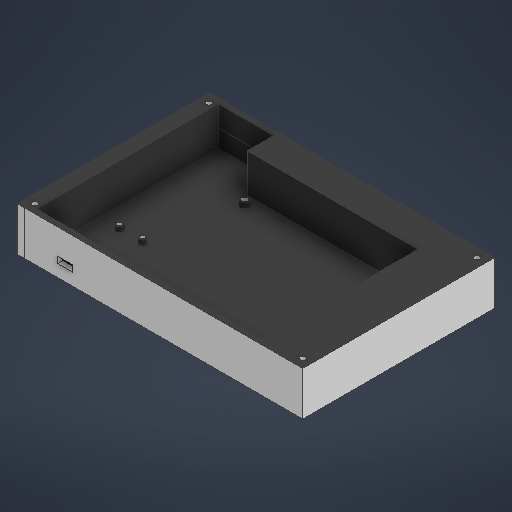
# Autodesk Inventor part: COC
Saved by Autodesk Inventor 2026 (Build 300175050, 175E)
## iProperties
Created: 2025-07-10
Part Number: COC
Material: Generic
Document SubType Name: Modeling
Designer: SaiAn
Density: 1 g/cm^3
Appearance: Default
Author: SaiAn
Autodesk Inventor part; units mm, degrees
ref_plane "YZ Plane" through (0, 0, 0) normal (1, 0, 0) x (0, 1, 0)
ref_plane "XZ Plane" through (0, 0, 0) normal (0, 1, 0) x (-1, 0, 0)
ref_plane "XY Plane" through (0, 0, 0) normal (0, 0, 1) x (1, 0, 0)
sketch "Sketch15" plane through (0, 0, 0) normal (0, 1, 0) x (-1, 0, 0)
  line L0 (0, 0) -> (97.63, 0)
  line L1 (97.63, 0) -> (97.63, -88.63)
  line L2 (97.63, -88.63) -> (0, -88.63)
  line L3 (0, -88.63) -> (0, 0)
  line L4 (-10, 10) -> (107.63, 10)
  line L5 (107.63, 10) -> (107.63, -98.63)
  line L6 (107.63, -98.63) -> (-10, -98.63)
  line L7 (-10, -98.63) -> (-10, 10)
  circle A0 centre (92.495, -6.851) radius 1.7
  circle A1 centre (93.005, -82.891) radius 1.7005
  circle A2 centre (4.245, -5.221) radius 1.7
  circle A3 centre (5.395, -84.151) radius 1.7
  circle A4 centre (92.495, -6.851) radius 2.5
  circle A5 centre (93.005, -82.891) radius 2.5
  circle A6 centre (4.245, -5.221) radius 2.5
  circle A7 centre (5.395, -84.151) radius 2.5
  dimension "d88" = 97.63
  dimension "d89" = 88.63
  dimension "d90" = 117.63
  dimension "d91" = 108.63
  dimension "d92" = 10
  dimension "d93" = 10
  dimension "d98" = 3.4
  dimension "d99" = 5.135
  dimension "d100" = 6.851
  dimension "d101" = 3.401
  dimension "d102" = 4.625
  dimension "d103" = 5.739
  dimension "d104" = 3.4
  dimension "d105" = 5.221
  dimension "d106" = 4.245
  dimension "d107" = 3.4
  dimension "d108" = 4.479
  dimension "d109" = 5.395
  dimension "d110" = 5
  dimension "d111" = 5
  dimension "d112" = 5
  dimension "d113" = 5
  constraints: 16 end point, 8 centre point, 4 coincident, 4 parallel, 2 horizontal, 2 perpendicular
  measures "d88" distance of L1.end L2.end
  measures "d89" distance of L0.end L1.end
  measures "d90" distance of L5.end L6.end
  measures "d91" distance of L4.end L5.end
  measures "d92" distance between parallel lines of L4 L0
  measures "d93" distance between parallel lines of L1 L5
  measures "d98" diameter of A0
  measures "d99" distance from line of L1 A0.centre
  measures "d100" distance from line of L0 A0.centre
  measures "d101" diameter of A1
  measures "d102" distance from line of L1 A1.centre
  measures "d103" distance from line of L2 A1.centre
  measures "d104" diameter of A2
  measures "d105" distance from line of L0 A2.centre
  measures "d106" distance from line of L3 A2.centre
  measures "d107" diameter of A3
  measures "d108" distance from line of L2 A3.centre
  measures "d109" distance from line of L3 A3.centre
  measures "d110" diameter of A4
  measures "d111" diameter of A5
  measures "d112" diameter of A6
  measures "d113" diameter of A7
extrude "Extrusion21" add sketch "Sketch15" along normal blind 3 contours L0 L1 L2 L3 | A0 | A1 | A2 | A3 | A4 | A5 | A6 | A7
extrude "Extrusion22" add sketch "Sketch15" along normal blind 13 contours L4 L5 L6 L7
extrude "Extrusion23" cut sketch "Sketch15" along normal blind 13 contours A0 | A1 | A2 | A3
extrude "Extrusion24" add sketch "Sketch15" along normal blind 6 contours A4 | A5 | A6 | A7
sketch "Sketch16" plane through (10, 0, -98.63) normal (0, 0, -1) x (-1, 0, 0)
  line L0 (0, 13) -> (117.63, 13) projected
  line L1 (117.63, 0) -> (0, 0) projected
  line L2 (117.63, 13) -> (0, 13)
  line L3 (0, 13) -> (0, 0)
  line L4 (0, 0) -> (117.63, 0)
  line L5 (117.63, 0) -> (117.63, 13)
  point P0 (10, 0)
  constraints: 8 end point, 2 parallel, 1 horizontal, 1 perpendicular
extrude "Extrusion25" add sketch "Sketch16" along normal blind 15.696
sketch "Sketch17" plane through (-97.63, 3, -88.63) normal (1, 0, 0) x (0, 0, -1)
  line L0 (0, 0) -> (0, 10) projected
  line L1 (-88.63, 10) -> (0, 10)
  line L2 (0, 10) -> (0, 0)
  line L3 (0, 0) -> (-88.63, 0)
  line L4 (-88.63, 0) -> (-88.63, 10)
  point P0 (-88.63, -3)
  constraints: 8 end point, 2 parallel, 1 horizontal, 1 perpendicular
extrude "Extrusion26" cut sketch "Sketch17" against normal blind 10
sketch "Sketch18" plane through (-107.63, 0, 10) normal (-1, 0, 0) x (0, 0, 1)
  line L0 (-98.63, 13) -> (-124.326, 13) projected
  line L1 (-124.326, 13) -> (-124.326, 0)
  line L2 (-124.326, 0) -> (0.0056, 0)
  line L3 (0.0056, 0) -> (0.0056, 13.0075)
  line L4 (0.0056, 13.0075) -> (-10, 13.0075)
  line L5 (-10, 13.0075) -> (-10, 3)
  line L6 (-98.63, 3) -> (-98.63, 13) projected
  line L7 (-10, 3) -> (-98.63, 3)
  line L8 (-98.63, 3) -> (-98.63, 13)
  point P0 (-10, 0)
  constraints: 14 end point, 6 perpendicular, 1 vertical
extrude "Extrusion27" add sketch "Sketch18" along normal blind 25
sketch "Sketch19" plane through (0, 3, 0) normal (0, 0, -1) x (-1, 0, 0)
  line L0 (107.63, 10.0075) -> (132.63, 10.0075) projected
  line L1 (132.63, 0) -> (0, 0) projected
  line L2 (132.63, 10.0075) -> (122.63, 10.0075)
  line L3 (122.63, 10.0075) -> (122.63, 0)
  line L4 (122.63, 0) -> (132.63, 0)
  line L5 (132.63, 0) -> (132.63, 10.0075)
  point P0 (0, -3)
  dimension "d124" = 10
  constraints: 8 end point, 2 parallel, 1 horizontal, 1 perpendicular, 1 point on line
  measures "d124" distance of L4.end L3.end
extrude "Extrusion28" add sketch "Sketch19" along normal blind 88.63
sketch "Sketch20" plane through (0, 3, 0) normal (0, 1, 0) x (1, 0, 0)
  circle A0 centre (-118.282, 3.585) radius 1.25
  line L0 (-107.63, 0) -> (-122.63, 0) projected
  line L1 (-122.63, 0) -> (-122.63, 88.63) projected
  circle A1 centre (-118.282, 3.585) radius 2
  circle A2 centre (-100.632, 3.585) radius 1.25
  circle A3 centre (-100.632, 3.585) radius 2
  circle A4 centre (-103.397, 35.123) radius 1.25
  line L2 (0, 0) -> (-107.63, 0) projected
  circle A5 centre (-116.397, 35.123) radius 1.25
  circle A6 centre (-103.397, 35.123) radius 2
  circle A7 centre (-116.397, 35.123) radius 2
  dimension "d127" = 2.5
  dimension "d128" = 3.585
  dimension "d129" = 4.348
  dimension "d130" = 4
  dimension "d131" = 2.5
  dimension "d132" = 3.585
  dimension "d133" = 21.998
  dimension "d134" = 4
  dimension "d135" = 2.5
  dimension "d136" = 19.233
  dimension "d137" = 35.123
  dimension "d138" = 2.5
  dimension "d139" = 6.233
  dimension "d140" = 35.123
  dimension "d141" = 4
  dimension "d142" = 4
  constraints: 8 centre point, 4 coincident
  measures "d127" diameter of A0
  measures "d128" distance from line of L0 A0.centre
  measures "d129" distance from line of L1 A0.centre
  measures "d130" diameter of A1
  measures "d131" diameter of A2
  measures "d132" distance from line of L0 A2.centre
  measures "d133" distance from line of L1 A2.centre
  measures "d134" diameter of A3
  measures "d135" diameter of A4
  measures "d136" distance from line of L1 A4.centre
  measures "d137" distance from line of L2 A4.centre
  measures "d138" diameter of A5
  measures "d139" distance from line of L1 A5.centre
  measures "d140" distance from line of L0 A5.centre
  measures "d141" diameter of A6
  measures "d142" diameter of A7
extrude "Extrusion29" add sketch "Sketch20" along normal blind 3
extrude "Extrusion30" cut sketch "Sketch20" against normal blind 6 contours A0 | A2 | A4 | A5
sketch "Sketch21" plane through (-122.63, 3, 0) normal (1, 0, 0) x (0, 0, -1)
  line L0 (88.63, 10) -> (88.63, 0) projected
  line L1 (0, 10.0075) -> (88.63, 10.0075) projected
  line L2 (88.63, 0) -> (0, 0)
  line L3 (0, 0) -> (0, 10.0075)
  line L4 (0, 10.0075) -> (88.63, 10.0075)
  line L5 (88.63, 10.0075) -> (88.63, 0)
  point P0 (0, -3)
  constraints: 8 end point, 2 parallel, 1 horizontal, 1 perpendicular
extrude "Extrusion31" cut sketch "Sketch21" against normal blind 6
sketch "Sketch22" plane through (0, 3, -88.63) normal (0, 0, 1) x (1, 0, 0)
  line L0 (0, 0) -> (-128.63, 0) projected
  line L1 (-128.63, 10) -> (0, 10) projected
  line L2 (-128.63, 0) -> (-97.315, 0)
  line L3 (-97.315, 0) -> (-97.315, 10)
  line L4 (-97.315, 10) -> (-128.63, 10)
  line L5 (-128.63, 10) -> (-128.63, 0)
  point P0 (0, -3)
  dimension "d149" = 31.315
  constraints: 8 end point, 2 parallel, 1 horizontal, 1 perpendicular, 1 point on line
  measures "d149" distance of L4.end L3.end
extrude "Extrusion32" cut sketch "Sketch22" against normal blind 15
sketch "Sketch23" plane through (10, 0, 10) normal (1, 0, 0) x (0, 0, -1)
  line L0 (0, 13) -> (10, 13) projected
  line L1 (124.326, 0) -> (-0.0056, 0) projected
  line L2 (0, 13) -> (124.326, 13)
  line L3 (124.326, 13) -> (124.326, 0)
  line L4 (124.326, 0) -> (0, 0)
  line L5 (0, 0) -> (0, 13)
  point P0 (10, 0)
  point P1 (0, 0)
  constraints: 8 end point, 2 parallel, 1 horizontal, 1 perpendicular
extrude "Extrusion33" add sketch "Sketch23" along normal blind 20
sketch "Sketch24" plane through (0, 13, 0) normal (0, 1, 0) x (1, 0, 0)
  line L0 (-107.63, -10) -> (30, -10) projected
  line L1 (30, 114.326) -> (14, 114.326)
  line L2 (14, 114.326) -> (14, -10)
  line L3 (14, -10) -> (30, -10)
  line L4 (30, -10) -> (30, 114.326)
  point P0 (0, 0)
  dimension "d154" = 16
  constraints: 8 end point, 2 parallel, 1 horizontal, 1 perpendicular, 1 point on line
  measures "d154" distance of L3.end L2.end
extrude "Extrusion34" add sketch "Sketch24" along normal blind 12
sketch "Sketch25" plane through (0, 13, 0) normal (0, 1, 0) x (1, 0, 0)
  line L0 (14, 114.326) -> (-132.63, 114.326) projected
  line L1 (-107.63, -10) -> (14, -10) projected
  line L2 (14, 114.326) -> (0, 114.326)
  line L3 (0, 114.326) -> (0, -10)
  line L4 (0, -10) -> (14, -10)
  line L5 (14, -10) -> (14, 114.326)
  line L6 (0, 88.63) -> (-97.315, 88.63) projected
  line L7 (0, 114.326) -> (-97.315, 114.326)
  line L8 (-97.315, 114.326) -> (-97.315, 88.63)
  line L9 (-97.315, 88.63) -> (0, 88.63)
  line L10 (0, 88.63) -> (0, 114.326)
  line L11 (0, 0) -> (-107.63, 0) projected
  line L12 (0, 0) -> (-132.63, 0)
  line L13 (-132.63, 0) -> (-132.63, -10)
  line L14 (-132.63, -10) -> (0, -10)
  line L15 (0, -10) -> (0, 0)
  line L16 (-107.63, 0) -> (-128.63, 0) projected
  line L17 (-128.63, 0) -> (-132.63, 0)
  line L18 (-132.63, 0) -> (-132.63, 114.326)
  line L19 (-132.63, 114.326) -> (-128.63, 114.326)
  line L20 (-128.63, 114.326) -> (-128.63, 0)
  line L21 (-97.315, 114.326) -> (-128.63, 114.326)
  line L22 (-128.63, 114.326) -> (-128.63, 103.6198)
  line L23 (-128.63, 103.6198) -> (-97.315, 103.6198)
  line L24 (-97.315, 103.6198) -> (-97.315, 114.326)
  point P0 (14, -10)
  constraints: 40 end point, 10 parallel, 5 horizontal, 5 perpendicular, 3 point on line
extrude "Extrusion35" add sketch "Sketch25" along normal blind 12 contours L5 L1 L3 L0 | L3 L6 L8 L0 | L8 L23 L20 L0 | L1 L14 L13 L12 L11 L3 | L20 L12 L18 L0
sketch "Sketch26" plane through (10, 0, -114.326) normal (0, 0, -1) x (-1, 0, 0)
  line L0 (-20, 0) -> (-20, 25) projected
  line L1 (-20, 0) -> (142.4813, 0)
  line L2 (142.4813, 0) -> (142.4813, 25)
  line L3 (142.4813, 25) -> (-20, 25)
  line L4 (-20, 25) -> (-20, 0)
  point P0 (10, 0)
  constraints: 8 end point, 2 parallel, 1 horizontal, 1 perpendicular
extrude "Extrusion36" cut sketch "Sketch26" against normal blind 8
sketch "Sketch27" plane through (-132.4813, 0, -114.326) normal (1, 0, 0) x (0, 0, -1)
  line L0 (0, 25) -> (-124.326, 25) projected
  line L1 (0, 0) -> (-7.9474, 0)
  line L2 (-7.9474, 0) -> (-7.9474, 25)
  line L3 (-7.9474, 25) -> (0, 25)
  line L4 (0, 25) -> (0, 0)
  point P0 (-114.326, 0)
  constraints: 8 end point, 2 parallel, 1 horizontal, 1 perpendicular, 1 point on line
extrude "Extrusion37" cut sketch "Sketch27" against normal blind 8
sketch "Sketch28" plane through (-132.63, 13.0075, 10) normal (0, 0, 1) x (1, 0, 0)
  line L0 (0, 11.9925) -> (162.63, 11.9925) projected
  line L1 (0.1487, -13.0075) -> (162.63, -13.0075) projected
  line L2 (0, 11.9925) -> (162.63, 11.9925)
  line L3 (162.63, 11.9925) -> (162.63, -13.0075)
  line L4 (162.63, -13.0075) -> (0, -13.0075)
  line L5 (0, -13.0075) -> (0, 11.9925)
  point P0 (132.63, -13.0075)
  constraints: 8 end point, 2 parallel, 1 horizontal, 1 perpendicular
extrude "Extrusion38" cut sketch "Sketch28" against normal blind 7
sketch "Sketch29" plane through (30, 0, 10) normal (1, 0, 0) x (0, 0, -1)
  line L0 (116.326, 0) -> (116.326, 25) projected
  line L1 (116.326, 0) -> (7, 0)
  line L2 (7, 0) -> (7, 25)
  line L3 (7, 25) -> (116.326, 25)
  line L4 (116.326, 25) -> (116.326, 0)
  point P0 (10, 0)
  constraints: 8 end point, 2 parallel, 1 horizontal, 1 perpendicular
extrude "Extrusion39" cut sketch "Sketch29" against normal blind 4
sketch "Sketch30" plane through (-132.63, 0, 10) normal (-1, 0, 0) x (0, 0, 1)
  line L0 (-116.326, 25) -> (-116.326, 0) projected
  line L1 (-116.326, 25) -> (-6.9664, 25)
  line L2 (-6.9664, 25) -> (-6.9664, 0)
  line L3 (-6.9664, 0) -> (-116.326, 0)
  line L4 (-116.326, 0) -> (-116.326, 25)
  point P0 (-10, 0)
  constraints: 8 end point, 2 parallel, 1 horizontal, 1 perpendicular
extrude "Extrusion40" add sketch "Sketch30" along normal blind 4
sketch "Sketch31" plane through (-107.63, 0, 10.0056) normal (0, 0, 1) x (1, 0, 0)
  line L0 (0, 13.0075) -> (-25, 13.0075) projected
  line L1 (-25, 13.0075) -> (0.1027, 13.0075)
  line L2 (0.1027, 13.0075) -> (0.1027, -0.1)
  line L3 (0.1027, -0.1) -> (-25, -0.1)
  line L4 (-25, -0.1) -> (-25, 13.0075)
  point P0 (107.63, 0)
  constraints: 8 end point, 2 parallel, 1 horizontal, 1 perpendicular
extrude "Extrusion41" cut sketch "Sketch31" against normal blind 1
sketch "Sketch33" plane through (0, 25, 0) normal (0, 1, 0) x (1, 0, 0)
  circle A0 centre (21, 101.326) radius 1.5
  circle A1 centre (21, 2) radius 1.5
  circle A2 centre (-131.63, 101.326) radius 1.5
  circle A3 centre (-131.63, 2) radius 1.5
  line L0 (-132.63, 106.326) -> (-136.63, 106.326) projected
  line L1 (-136.63, -3.0336) -> (-136.63, 106.326) projected
  line L2 (-132.63, -3) -> (26, -3) projected
  line L3 (26, -3) -> (26, 106.326) projected
  line L4 (26, 106.326) -> (-132.4813, 106.326) projected
  point P0 (0, 0)
  dimension "d171" = 3
  dimension "d172" = 3
  dimension "d173" = 3
  dimension "d174" = 3
  dimension "d175" = 5
  dimension "d176" = 5
  dimension "d177" = 5
  dimension "d178" = 5
  dimension "d179" = 5
  dimension "d180" = 5
  dimension "d181" = 5
  dimension "d182" = 5
  constraints: 4 centre point
  measures "d171" diameter of A0
  measures "d172" diameter of A1
  measures "d173" diameter of A2
  measures "d174" diameter of A3
  measures "d175" distance from line of L0 A2.centre
  measures "d176" distance from line of L1 A2.centre
  measures "d177" distance from line of L1 A3.centre
  measures "d178" distance from line of L2 A3.centre
  measures "d179" distance from line of L3 A0.centre
  measures "d180" distance from line of L4 A0.centre
  measures "d181" distance from line of L2 A1.centre
  measures "d182" distance from line of L3 A1.centre
extrude "Extrusion42" cut sketch "Sketch33" against normal blind 25
sketch "Sketch34" plane through (0, 0, 0) normal (0, -1, 0) x (1, 0, 0)
  circle A0 centre (21, -2) radius 1.5 projected
  circle A1 centre (21, -2) radius 3
  circle A2 centre (21, -101.326) radius 1.5 projected
  circle A3 centre (21, -101.326) radius 3
  circle A4 centre (-131.63, -2) radius 1.5 projected
  circle A5 centre (-131.63, -2) radius 3
  circle A6 centre (-131.63, -101.326) radius 1.5 projected
  circle A7 centre (-131.63, -101.326) radius 3
  point P0 (0, 0)
  dimension "d185" = 6
  dimension "d186" = 6
  dimension "d187" = 6
  dimension "d188" = 6
  constraints: 4 centre point, 4 coincident
  measures "d185" diameter of A1
  measures "d186" diameter of A3
  measures "d187" diameter of A5
  measures "d188" diameter of A7
extrude "Extrusion43" cut sketch "Sketch34" against normal blind 5 contours A0 | A1 | A2 | A3 | A4 | A5 | A6 | A7
sketch "Sketch35" plane through (-132.63, 13.0075, 3) normal (0, 0, 1) x (1, 0, 0)
  line L0 (27.657, -2.4225) -> (18.992, -2.4225)
  line L1 (18.992, -2.4225) -> (18.992, -6.0255)
  line L2 (18.992, -6.0255) -> (27.657, -6.0255)
  line L3 (27.657, -6.0255) -> (27.657, -2.4225)
  line L4 (-4, -13.0075) -> (-4, 11.9925) projected
  line L5 (158.63, -13.0075) -> (0, -13.0075) projected
  point P0 (132.63, -13.0075)
  dimension "d191" = 8.665
  dimension "d192" = 3.603
  dimension "d193" = 22.992
  dimension "d197" = 6.982
  constraints: 8 end point, 2 parallel, 1 horizontal, 1 perpendicular
  measures "d191" distance of L2.end L1.end
  measures "d192" distance of L1.end L0.end
  measures "d193" distance between parallel lines of L4 L1
  measures "d197" distance between parallel lines of L2 L5
extrude "Extrusion44" cut sketch "Sketch35" against normal blind 10
body "Solid2"
